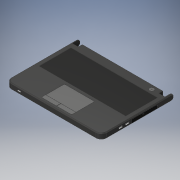
# Autodesk Inventor part: BOARD
Saved by Autodesk Inventor 2025 (Build 290162000, 162)
## iProperties
Created: 2017-02-17
Part Number: BOARD
Material: Generic
Document SubType Name: Modeling
Designer: Ali
Density: 1 g/cm^3
Appearance: Default
Author: Ali
Autodesk Inventor part; units mm, degrees
ref_plane "YZ Plane" through (0, 0, 0) normal (1, 0, 0) x (0, 1, 0)
ref_plane "XZ Plane" through (0, 0, 0) normal (0, 1, 0) x (-1, 0, 0)
ref_plane "XY Plane" through (0, 0, 0) normal (0, 0, 1) x (1, 0, 0)
sketch "Sketch1" plane through (0, 0, 0) normal (0, 1, 0) x (-1, 0, 0)
  line L0 (-165, -250) -> (-165, -20)
  line L1 (-145, 0) -> (145, 0)
  line L2 (165, -20) -> (165, -250)
  arc A0 (165, -20) -> (145, 0) centre (145, -20) ccw
  arc A1 (-145, 0) -> (-165, -20) centre (-145, -20) ccw
  line L3 (-139.5, -228) -> (-160.5, -228)
  line L4 (-160.5, -228) -> (-160.5, -250)
  line L5 (-160.5, -250) -> (-165, -250)
  line L6 (-139.5, -228) -> (-139.5, -239)
  line L7 (-139.5, -239) -> (139.5, -239)
  line L8 (139.5, -239) -> (139.5, -228)
  line L9 (139.5, -228) -> (160.5, -228)
  line L10 (160.5, -228) -> (160.5, -250)
  line L11 (160.5, -250) -> (165, -250)
  point P0 (-165, 0)
  point P1 (165, 0)
  dimension "d19" = 279
  dimension "d20" = 11
  dimension "d21" = 21
  dimension "d22" = 22
  constraints: 24 end point, 4 point on circle, 4 point on line, 4 tangent, 2 centre point, 1 equal radius, 1 parallel
  measures "d19" distance of L6.end L7.end
  measures "d20" distance of L3.start L6.end
  measures "d21" distance of L3.end L3.start
  measures "d22" distance of L4.end L3.end
extrude "BOARD" add sketch "Sketch1" along normal blind 20
chamfer "HINGE CHAMFER" distance 2.5 angle 45 4 edges at (-150, 20, -228) (150, 20, -228) (150, 0, -228) (-150, 0, -228)
sketch "Sketch2" plane through (0, 20, 0) normal (0, 1, 0) x (1, 0, 0)
  line L0 (-47.5, 10) -> (47.5, 10)
  line L1 (52.5, 15) -> (52.5, 85)
  line L2 (47.5, 90) -> (-47.5, 90)
  line L3 (-52.5, 85) -> (-52.5, 15)
  arc A0 (-47.5, 90) -> (-52.5, 85) centre (-47.5, 85) ccw
  arc A1 (52.5, 85) -> (47.5, 90) centre (47.5, 85) ccw
  arc A2 (47.5, 10) -> (52.5, 15) centre (47.5, 15) ccw
  arc A3 (-52.5, 15) -> (-47.5, 10) centre (-47.5, 15) ccw
  point P0 (52.5, 90)
  point P1 (52.5, 10)
  point P2 (-52.5, 90)
  dimension "d32" = 105
  dimension "d33" = 80
  dimension "d34" = 5
  constraints: 8 end point, 8 point on circle, 8 tangent, 6 point on line, 4 centre point, 3 equal radius, 2 parallel, 1 horizontal, 1 perpendicular
  measures "d32" distance of point (-52.5, 90) point (52.5, 90)
  measures "d33" distance of point (52.5, 90) point (52.5, 10)
  measures "d34" radius of A0
extrude "TOUCH PAD" cut sketch "Sketch2" against normal blind 0.5
sketch "Sketch3" plane through (0, 19.5, 0) normal (0, 1, 0) x (1, 0, 0)
  line L0 (-52.5, 25) -> (-0.5, 25)
  line L1 (-0.5, 25) -> (-0.5, 10)
  line L2 (-0.5, 10) -> (-47.5, 10)
  line L3 (-52.5, 15) -> (-52.5, 25)
  arc A0 (-52.5, 15) -> (-47.5, 10) centre (-47.5, 15) ccw
  point P0 (-52.5, 10)
  dimension "d39" = 52
  dimension "d40" = 15
  dimension "d41" = 5
  constraints: 8 end point, 2 parallel, 2 point on circle, 2 point on line, 2 tangent, 1 centre point, 1 horizontal, 1 perpendicular
  measures "d39" distance of L1.end point (-52.5, 10)
  measures "d40" distance of L0.end L1.end
  measures "d41" radius of A0
extrude "LEFT BUTTON" add sketch "Sketch3" along normal blind 0.6
sketch "Sketch4" plane through (0, 19.5, 0) normal (0, 1, 0) x (1, 0, 0)
  line L0 (0.5, 25) -> (52.5, 25)
  line L1 (52.5, 25) -> (52.5, 15)
  line L2 (47.5, 10) -> (0.5, 10)
  line L3 (0.5, 10) -> (0.5, 25)
  arc A0 (47.5, 10) -> (52.5, 15) centre (47.5, 15) ccw
  constraints: 8 end point, 2 parallel, 2 point on circle, 2 tangent, 1 centre point, 1 horizontal, 1 perpendicular
extrude "RIGHT BUTTON" add sketch "Sketch4" along normal blind 0.6
sketch "Sketch5" plane through (0, 20, 0) normal (0, 1, 0) x (1, 0, 0)
  line L0 (-150, 210) -> (150, 210)
  line L1 (150, 210) -> (150, 100)
  line L2 (150, 100) -> (-150, 100)
  line L3 (-150, 100) -> (-150, 210)
  dimension "d57" = 300
  dimension "d58" = 110
  constraints: 8 end point, 2 parallel, 1 horizontal, 1 perpendicular
  measures "d57" distance of L1.end L2.end
  measures "d58" distance of L0.end L1.end
extrude "KEYBOARD BASE" cut sketch "Sketch5" against normal blind 0.3
chamfer "KEYBOARD CHAMFER" distance 0.3 angle 45 4 edges at (-150, 20, -155) (0, 20, -100) (0, 20, -210) (150, 20, -155)
sketch "Sketch6" plane through (165, 0, -20) normal (1, 0, 0) x (0, 0, -1)
  line L0 (230, 20) -> (222.0031, 20)
  line L1 (222.0031, 20) -> (222.0031, 0)
  line L2 (222.0031, 0) -> (230, 0)
  line L3 (230, 0) -> (230, 20)
  point P0 (-20, 0)
  constraints: 8 end point, 2 parallel, 1 horizontal, 1 perpendicular
extrude "CUT" cut sketch "Sketch6" against normal blind 330
sketch "Sketch7" plane through (165, 0, -20) normal (1, 0, 0) x (0, 0, -1)
  arc A0 (222.0031, 0) -> (222.0031, 20) centre (222.0031, 10) ccw
  line L0 (222.0031, 20) -> (222.0031, 0)
  point P0 (-20, 0)
  constraints: 2 end point, 2 point on circle, 1 centre point
extrude "ROUND BASE" add sketch "Sketch7" against normal blind 4.5
sketch "Sketch8" plane through (-165, 0, -20) normal (-1, 0, 0) x (0, 0, 1)
  arc A0 (-222.0031, 20) -> (-222.0031, 0) centre (-222.0031, 10) ccw
  line L0 (-222.0031, 20) -> (-222.0031, 0)
  point P0 (20, 0)
  constraints: 2 end point, 2 point on circle, 1 centre point
extrude "ROUND BASE 1" add sketch "Sketch8" against normal blind 4.5
chamfer "BOARD BASE" distance 2.5 angle 45 12 edges at (165, 0, -131.0016) (159.1421, 0, -5.8579) (0, 0, 0) (-159.1421, 0, -5.8579) (-165, 0, -131.0016) (-165, 10, -252.0031) (-165, 20, -131.0016) (-159.1421, 20, -5.8579) (0, 20, 0) (159.1421, 20, -5.8579) (165, 20, -131.0016) (165, 10, -252.0031)
sketch "Sketch9" plane through (0, 20, 0) normal (0, 1, 0) x (1, 0, 0)
  circle A0 centre (115, 225) radius 7.5
  point P0 (0, 0)
  dimension "d73" = 15
  constraints: 1 centre point
  measures "d73" diameter of A0
extrude "POWER BUTTON" cut sketch "Sketch9" against normal blind 0.05
sketch "Sketch10" plane through (115, 19.95, -225) normal (0, 1, 0) x (1, 0, 0)
  point P0 (-115, -225)
  point P1 (0, 0)
hole "POWER BUTTON 1" at (115, 19.95, -225) direction (0, -1, 0) diameter 2 depth 0.05 tip angle 118
sketch "Sketch11" plane through (-165, 10, -242.0031) normal (-1, 0, 0) x (0, 0, 1)
  point P0 (242.0031, -10)
  point P1 (25, 0)
hole "CHARGING PORT" at (-165, 10, -217.0031) direction (1, 0, 0) diameter 6.5 depth 5.1 counterbore diameter 8.5 counterbore depth 0.1
sketch "Sketch12" plane through (-165, 10, -242.0031) normal (-1, 0, 0) x (0, 0, 1)
  line L0 (56.5, 4) -> (56.5, -4)
  line L1 (55, 4) -> (55, -4)
  arc A0 (56.5, 4) -> (55, 4) centre (55.75, 4) ccw
  arc A1 (55, -4) -> (56.5, -4) centre (55.75, -4) ccw
  point P0 (242.0031, -10)
  constraints: 4 end point, 4 point on circle, 2 centre point
extrude "HEAT SINK" cut sketch "Sketch12" against normal blind 2
pattern_linear "HEAT SINK PATTERN" count 15 spacing 4 along (0, 0, 1) of "HEAT SINK"
sketch "Sketch13" plane through (-165, 10, -242.0031) normal (-1, 0, 0) x (0, 0, 1)
  line L0 (120, 3) -> (133, 3)
  line L1 (133, -3) -> (131.3617, -4.1472)
  line L2 (133, 3) -> (133, -3)
  line L3 (120, 3) -> (120, -3)
  line L4 (120, -3) -> (121.6383, -4.1472)
  line L5 (121.6383, -4.1472) -> (131.3617, -4.1472)
  constraints: 12 end point
extrude "HDMI PORT" cut sketch "Sketch13" against normal blind 5
sketch "Sketch14" plane through (-160, 10, -242.0031) normal (-1, 0, 0) x (0, 0, 1)
  line L0 (120.3048, -1) -> (132.7049, -1)
  line L1 (132.7049, -1) -> (132.7049, -1.5)
  line L2 (132.7049, -1.5) -> (120.3048, -1.5)
  line L3 (120.3048, -1.5) -> (120.3048, -1)
  point P0 (242.0031, -10)
  constraints: 8 end point, 2 parallel, 1 horizontal, 1 perpendicular
extrude "HDMI SLOT" add sketch "Sketch14" along normal blind 5
sketch "Sketch15" plane through (-165, 10, -242.0031) normal (-1, 0, 0) x (0, 0, 1)
  line L0 (158, -3) -> (145, -3)
  line L1 (145, -3) -> (145, 3)
  line L2 (145, 3) -> (158, 3)
  line L3 (158, 3) -> (158, -3)
  constraints: 8 end point, 2 parallel, 1 horizontal, 1 perpendicular
extrude "USB PORT" cut sketch "Sketch15" against normal blind 5
sketch "Sketch16" plane through (-160, 10, -242.0031) normal (-1, 0, 0) x (0, 0, 1)
  line L0 (145.3, 1.5) -> (157.7, 1.5)
  line L1 (157.7, 1.5) -> (157.7, 1)
  line L2 (157.7, 1) -> (145.3, 1)
  line L3 (145.3, 1) -> (145.3, 1.5)
  point P0 (242.0031, -10)
  dimension "d126" = 12.4
  dimension "d127" = 0.5
  constraints: 8 end point, 2 parallel, 1 horizontal, 1 perpendicular
  measures "d126" distance of L1.end L2.end
  measures "d127" distance of L0.end L1.end
extrude "USB SLOT" add sketch "Sketch16" along normal blind 5
sketch "Sketch17" plane through (-165, 10, -242.0031) normal (-1, 0, 0) x (0, 0, 1)
  line L0 (207.5, -2.5) -> (172.5, -2.5)
  line L1 (170, 0) -> (170, 0)
  line L2 (172.5, 2.5) -> (207.5, 2.5)
  line L3 (210, 0) -> (210, 0)
  arc A0 (210, 0) -> (207.5, 2.5) centre (207.5, 0) ccw
  arc A1 (207.5, -2.5) -> (210, 0) centre (207.5, 0) ccw
  arc A2 (172.5, 2.5) -> (170, 0) centre (172.5, 0) ccw
  arc A3 (170, 0) -> (172.5, -2.5) centre (172.5, 0) ccw
  point P0 (210, -2.5)
  point P1 (170, 2.5)
  point P2 (210, 2.5)
  dimension "d134" = 40
  dimension "d136" = 5
  dimension "d137" = 2.5
  constraints: 8 end point, 8 point on circle, 8 tangent, 6 point on line, 4 centre point, 3 equal radius, 2 parallel, 1 horizontal, 1 perpendicular
  measures "d134" distance of point (170, 2.5) point (210, 2.5)
  measures "d136" distance of point (210, 2.5) point (210, -2.5)
  measures "d137" radius of A0
extrude "MEMORY SLOT" cut sketch "Sketch17" against normal blind 5
sketch "Sketch18" plane through (165, 10, -242.0031) normal (1, 0, 0) x (0, 0, -1)
  line L0 (-132.5, 5.1) -> (-52.5, 5.1)
  line L1 (-47.5, 0.1) -> (-47.5, -7.4)
  line L2 (-47.5, -7.4) -> (-137.5, -7.4)
  line L3 (-137.5, -7.4) -> (-137.5, 0.1)
  arc A0 (-132.5, 5.1) -> (-137.5, 0.1) centre (-132.5, 0.1) ccw
  arc A1 (-47.5, 0.1) -> (-52.5, 5.1) centre (-52.5, 0.1) ccw
  point P0 (-47.5, 5.1)
  dimension "d147" = 5
  dimension "d148" = 12.5
  dimension "d150" = 90
  constraints: 8 end point, 4 point on circle, 4 tangent, 2 centre point, 2 parallel, 2 point on line, 1 horizontal, 1 perpendicular
  measures "d147" radius of A0
  measures "d148" distance of point (-47.5, 5.1) L1.end
  measures "d150" distance of L1.end L2.end
extrude "DISK HOLDER" add sketch "Sketch18" along normal blind 0.2
sketch "Sketch19" plane through (165.2, 10, -242.0031) normal (1, 0, 0) x (0, 0, -1)
  line L0 (-94, 1.6) -> (-98, 1.6)
  line L1 (-98.5, 1.1) -> (-98.5, 0.6)
  line L2 (-98, 0.1) -> (-94, 0.1)
  line L3 (-93.5, 0.6) -> (-93.5, 1.1)
  arc A0 (-98, 1.6) -> (-98.5, 1.1) centre (-98, 1.1) ccw
  arc A1 (-98.5, 0.6) -> (-98, 0.1) centre (-98, 0.6) ccw
  arc A2 (-94, 0.1) -> (-93.5, 0.6) centre (-94, 0.6) ccw
  arc A3 (-93.5, 1.1) -> (-94, 1.6) centre (-94, 1.1) ccw
  point P0 (-242.0031, -10)
  point P1 (-93.5, 1.6)
  point P2 (-98.5, 1.6)
  point P3 (-93.5, 0.1)
  dimension "d158" = 5
  dimension "d159" = 1.5
  dimension "d160" = 0.5
  constraints: 8 end point, 8 point on circle, 8 tangent, 6 point on line, 4 centre point, 3 equal radius, 2 parallel, 1 horizontal, 1 perpendicular
  measures "d158" distance of point (-93.5, 1.6) point (-98.5, 1.6)
  measures "d159" distance of point (-93.5, 0.1) point (-93.5, 1.6)
  measures "d160" radius of A0
extrude "DISK HOLDER BUTTON" add sketch "Sketch19" along normal blind 0.05
sketch "Sketch22" plane through (165, 10.0137, 60.9943) normal (1, 0, 0) x (0, 0, -1)
  line L0 (158, -3) -> (145, -3)
  line L1 (145, -3) -> (145, 3)
  line L2 (145, 3) -> (158, 3)
  line L3 (158, 3) -> (158, -3)
  constraints: 8 end point, 2 parallel, 1 horizontal, 1 perpendicular
extrude "USB PORT 1" cut sketch "Sketch22" against normal blind 5
sketch "Sketch23" plane through (160, 10.0137, 60.9943) normal (1, 0, 0) x (0, 0, -1)
  line L0 (145.3, 1.5) -> (157.7, 1.5)
  line L1 (157.7, 1.5) -> (157.7, 1)
  line L2 (157.7, 1) -> (145.3, 1)
  line L3 (145.3, 1) -> (145.3, 1.5)
  point P0 (242.0031, -10)
  dimension "d174" = 12.4
  dimension "d175" = 0.5
  constraints: 8 end point, 2 parallel, 1 horizontal, 1 perpendicular
  measures "d174" distance of L1.end L2.end
  measures "d175" distance of L0.end L1.end
extrude "USB SLOT 1" add sketch "Sketch23" along normal blind 5
sketch "Sketch24" plane through (165, 9.9349, 84.1739) normal (1, 0, 0) x (0, 0, -1)
  line L0 (158, -3) -> (145, -3)
  line L1 (145, -3) -> (145, 3)
  line L2 (145, 3) -> (158, 3)
  line L3 (158, 3) -> (158, -3)
  constraints: 8 end point, 2 parallel, 1 horizontal, 1 perpendicular
extrude "USB PORT 2" cut sketch "Sketch24" against normal blind 5
sketch "Sketch25" plane through (160, 9.9349, 84.1739) normal (1, 0, 0) x (0, 0, -1)
  line L0 (145.3, 1.5) -> (157.7, 1.5)
  line L1 (157.7, 1.5) -> (157.7, 1)
  line L2 (157.7, 1) -> (145.3, 1)
  line L3 (145.3, 1) -> (145.3, 1.5)
  point P0 (242.0031, -10)
  dimension "d182" = 12.4
  dimension "d183" = 0.5
  constraints: 8 end point, 2 parallel, 1 horizontal, 1 perpendicular
  measures "d182" distance of L1.end L2.end
  measures "d183" distance of L0.end L1.end
extrude "USB SLOT 2" add sketch "Sketch25" along normal blind 5
sketch "Sketch26" plane through (-145, 17.5, 0) normal (0, 0, 1) x (1, 0, 0)
  line L0 (22, -5.5) -> (30, -5.5)
  line L1 (32, -7.5) -> (32, -7.5)
  line L2 (30, -9.5) -> (22, -9.5)
  line L3 (20, -7.5) -> (20, -7.5)
  arc A0 (22, -5.5) -> (20, -7.5) centre (22, -7.5) ccw
  arc A1 (20, -7.5) -> (22, -9.5) centre (22, -7.5) ccw
  arc A2 (30, -9.5) -> (32, -7.5) centre (30, -7.5) ccw
  arc A3 (32, -7.5) -> (30, -5.5) centre (30, -7.5) ccw
  point P0 (145, -17.5)
  point P1 (32, -9.5)
  point P2 (32, -5.5)
  point P3 (20, -9.5)
  dimension "d190" = 12
  dimension "d191" = 4
  dimension "d192" = 2
  constraints: 8 end point, 8 point on circle, 8 tangent, 6 point on line, 4 centre point, 3 equal radius, 2 parallel, 1 horizontal, 1 perpendicular
  measures "d190" distance of point (32, -9.5) point (20, -9.5)
  measures "d191" distance of point (32, -5.5) point (32, -9.5)
  measures "d192" radius of A0
extrude "BATTERY INDICATOR" add sketch "Sketch26" along normal blind 0.05
body "Solid1"
